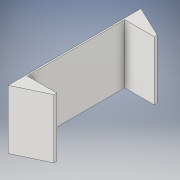
# Autodesk Inventor part: MAN_BASIS_GRIPPER
Saved by Autodesk Inventor 2019 (Build 230136000, 136)
## iProperties
Created: 2021-03-07
Part Number: MAN_BASIS_GRIPPER
Material: ABS Plastic
Document SubType Name: Modeling
Designer: DOMEK
Density: 1.06 g/cm^3
Appearance: Smooth - White
Author: DOMEK
Autodesk Inventor part; units mm, degrees
ref_plane "YZ Plane" through (0, 0, 0) normal (1, 0, 0) x (0, 1, 0)
ref_plane "XZ Plane" through (0, 0, 0) normal (0, 1, 0) x (-1, 0, 0)
ref_plane "XY Plane" through (0, 0, 0) normal (0, 0, 1) x (1, 0, 0)
sketch "Sketch1" plane through (0, 0, 0) normal (1, 0, 0) x (0, 1, 0)
  line L0 (0, 0) -> (40, 0)
  line L1 (40, 0) -> (40, 70)
  line L2 (40, 70) -> (0, 70)
  line L3 (0, 70) -> (0, 0)
  dimension "d0" = 40
  dimension "d1" = 70
  constraints: 8 end point, 2 parallel, 1 horizontal, 1 perpendicular
  measures "d0" distance of L2.end L1.end
  measures "d1" distance of L1.end L0.end
extrude "Extrusion1" add sketch "Sketch1" along normal blind 1
sketch "Sketch2" plane through (1, 0, 0) normal (1, 0, 0) x (0, 0, -1)
  line L0 (-70, 40) -> (-70, 0) projected
  line L1 (-70, 0) -> (0, 0) projected
  line L2 (-70, 40) -> (-68, 40)
  line L3 (-68, 40) -> (-68, 0)
  line L4 (-68, 0) -> (-70, 0)
  line L5 (-70, 0) -> (-70, 40)
  line L6 (0, 0) -> (0, 40) projected
  line L7 (0, 40) -> (-2, 40)
  line L8 (-2, 40) -> (-2, 0)
  line L9 (-2, 0) -> (0, 0)
  line L10 (0, 0) -> (0, 40)
  dimension "d4" = 2
  dimension "d5" = 2
  constraints: 16 end point, 4 parallel, 2 horizontal, 2 perpendicular, 2 point on line
  measures "d4" distance of L3.end L4.end
  measures "d5" distance of L9.end L8.end
extrude "Extrusion2" add sketch "Sketch2" along normal blind 20
sketch "Sketch4" plane through (0, 40, 70) normal (0, 1, 0) x (1, 0, 0)
  line L0 (0, 70) -> (0, 80)
  line L1 (21, 68) -> (21, 70) projected
  line L2 (0, 80) -> (21, 70)
  line L3 (0, 70) -> (0, 0) projected
  line L4 (0, 0) -> (0, -10)
  line L5 (0, 0) -> (21, 0) projected
  line L6 (0, -10) -> (21, 0)
  line L7 (0, 70) -> (21, 70)
  line L8 (1, 68) -> (21, 68) projected
  dimension "d8" = 10
  dimension "d9" = 10
  constraints: 10 end point, 2 vertical, 1 parallel
  measures "d8" distance of L0.start L0.end
  measures "d9" distance of L3.end L4.end
extrude "Extrusion3" add sketch "Sketch4" against normal blind 40
body "Solid1"
